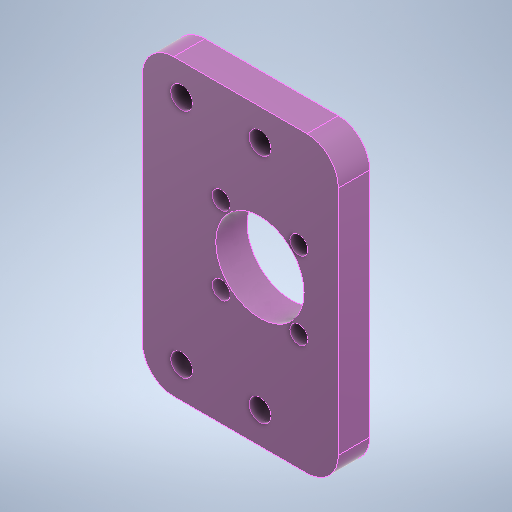
# Autodesk Inventor part: кронштейн
Saved by Autodesk Inventor 2025 (Build 290162000, 162)
## iProperties
Created: 2025-02-17
Part Number: кронштейн
Material: Сталь
Document SubType Name: Sheet Metal
Designer: volko
Density: 7.85 g/cm^3
Sheet Metal Rule: По умолчанию_мм
Appearance: Гладкий — пурпурный
Mass: 145.221 g
Surface Area: 142.245 cm^2
Volume: 18.4995 cm^3
Author: volko
Autodesk Inventor part; units mm, degrees
ref_plane "YZ Plane" through (0, 0, 0) normal (1, 0, 0) x (0, 1, 0)
ref_plane "XZ Plane" through (0, 0, 0) normal (0, 1, 0) x (-1, 0, 0)
ref_plane "XY Plane" through (0, 0, 0) normal (0, 0, 1) x (1, 0, 0)
sketch "Эскиз1" plane through (0, 0, 0) normal (0, 0, 1) x (1, 0, 0)
  line L0 (-1.5933, 37.5) -> (12, 37.5)
  line L1 (20, 29.5) -> (20, -29.5)
  arc A0 (20, 29.5) -> (12, 37.5) centre (12, 29.5) ccw
  line L2 (-1.5933, 37.5) -> (-22, 37.5)
  line L3 (-30, 29.5) -> (-30, -29.5)
  arc A1 (-22, 37.5) -> (-30, 29.5) centre (-22, 29.5) ccw
  line L4 (-42.3196, 0) -> (32.3196, 0) projected
  line L5 (0, -54.8196) -> (0, 54.8196) projected
  circle A2 centre (0, 2) radius 11.25
  circle A3 centre (0, 2) radius 14 construction
  line L6 (0, 2) -> (-9.8995, 11.8995) construction
  line L7 (-22, -37.5) -> (12, -37.5)
  arc A4 (-30, -29.5) -> (-22, -37.5) centre (-22, -29.5) ccw
  arc A5 (12, -37.5) -> (20, -29.5) centre (12, -29.5) ccw
  line L8 (0, 29.5) -> (-20, 29.5) construction
  line L9 (0, -29.5) -> (-20, -29.5) construction
  point P0 (0, 0)
  point P1 (0, 0)
  point P2 (0, 54.8196)
  point P3 (9.8995, 11.8995)
  point P4 (-9.8995, -7.8995)
  point P5 (9.8995, -7.8995)
  point P6 (20, 0)
  dimension "d128" = 28
  dimension "d43" = 8
  dimension "d50" = 20
  dimension "d127" = 22.5
  dimension "d131" = 360
  dimension "d134" = 45
  dimension "d168" = 8
  dimension "d182" = 2
  dimension "d200" = 20
  dimension "d201" = 50
  dimension "d202" = 75
  constraints: 16 end point, 8 point on circle, 8 tangent, 5 centre point, 3 equal radius, 3 horizontal, 2 symmetric about line, 1 coincident, 1 midpoint, 1 perpendicular, 1 point on line, 12 other
  measures "d43" radius of A0
  measures "d50" distance of L8.start L8.end
  measures "d127" diameter of A2
  measures "d134" angle of L6 L4
  measures "d168" distance from line of L0 L8.start
  measures "d182" distance from line of L4 L6.start
  measures "d200" distance of the line from the sketch origin of L1
  measures "d201" distance between parallel lines of L1 L3
  measures "d202" distance between parallel lines of L7 L2
extrude "Пластина2" add sketch "Эскиз1" along normal blind 8 contours L0 L5 A2 L4 L3 A1 L2 | L0 A0 L1 L4 A2 L5 | A2 L5 L7 A4 L3 L4 | L1 A5 L7 L5 A2 L4
hole "Отверстие2" at (-20, 29.5, 0) at (0, 29.5, 0) at (0, -29.5, 0) at (-20, -29.5, 0) direction (0, 0, 1) diameter 5.5 end through all countersink diameter 10.5 countersink angle 90
sketch "Эскиз6" plane through (0, 0, 8) normal (0, 0, 1) x (1, 0, 0)
  circle A0 centre (0, 2) radius 14 construction
  line L0 (0, -54.8196) -> (0, 54.8196) projected
  line L1 (-42.3196, 0) -> (32.3196, 0) projected
  line L2 (0, 2) -> (9.8995, 11.8995) construction
  point P0 (-9.8995, 11.8995)
  point P1 (-9.8995, -7.8995)
  point P2 (9.8995, -7.8995)
  dimension "d135" = 28
  dimension "d138" = 360
  dimension "d141" = 135
  dimension "d183" = 2
  constraints: 2 end point, 1 point on line, 8 other
  measures "d141" angle of L2 L1
  measures "d183" distance from line of L1 L2.start
hole "Отверстие3" at (-9.8995, -7.8995, 8) at (9.8995, 11.8995, 8) at (-9.8995, 11.8995, 8) at (9.8995, -7.8995, 8) direction (0, 0, -1) diameter 4.5 end through all
equation "\"d18\" = Толщина"
equation "\"Радиус_гибки\" = Толщина"
equation "\"Ширина_просечки\" = Толщина"
equation "\"Глубина_просечки\" = 0.5 * Толщина"
equation "\"Размер_просечки\" = 4 * Толщина"
equation "\"Мин_остаток\" = 2 * Толщина"
equation "\"Радиус_перехода\" = Радиус_гибки"
equation "\"Радиус_Якоби\" = Радиус_гибки"
equation "\"Размер_зазора\" = Толщина"
equation "\"Толщина\" = 8"
